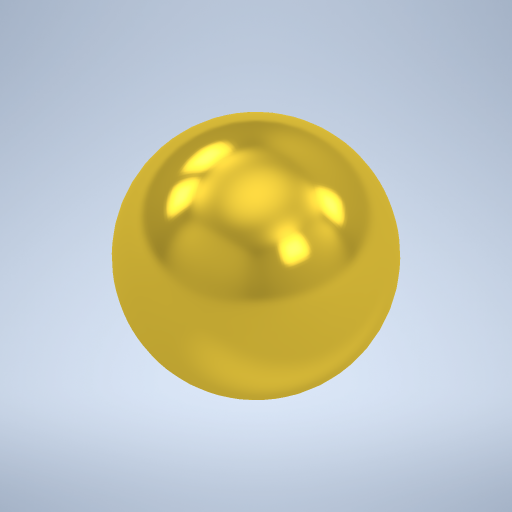
# Autodesk Inventor part: ball
Saved by Autodesk Inventor 2023 (Build 270158000, 158)
## iProperties
Created: 2023-03-23
Part Number: ball
Material: Generic
Document SubType Name: Modeling
Designer: CASPER
Density: 1 g/cm^3
Appearance: Metal 2400F Hot
Author: CASPER
Autodesk Inventor part; units mm, degrees
ref_plane "YZ Plane" through (0, 0, 0) normal (1, 0, 0) x (0, 1, 0)
ref_plane "XZ Plane" through (0, 0, 0) normal (0, 1, 0) x (-1, 0, 0)
ref_plane "XY Plane" through (0, 0, 0) normal (0, 0, 1) x (1, 0, 0)
sketch "Sketch1" plane through (0, 0, 0) normal (0, 0, 1) x (1, 0, 0)
  arc A0 (1.2, 0) -> (-1.2, 0) centre (0, 0) ccw
  line L0 (-1.2, 0) -> (1.2, 0)
  dimension "d0" = 2.4
  dimension "d1" = 1.2
  dimension "d2" = 2.4
  constraints: 2 end point, 2 point on circle, 1 centre point, 1 coincident
  measures "d0" diameter of A0
  measures "d1" radius of A0
  measures "d2" distance of L0.start L0.end
revolve "Revolution1" add sketch "Sketch1" angle 360 about axis through (-1.2, 0, 0) along (1, 0, 0)
body "Solid1"
